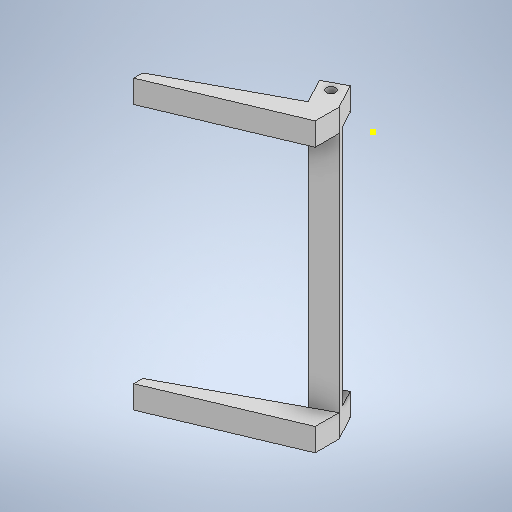
# Autodesk Inventor part: Part8
Saved by Autodesk Inventor 2025.2 (Build 292293000, 293)
## iProperties
Created: 2025-06-06
Part Number: Part8
Material: Generic
Document SubType Name: Sheet Metal
Designer: ziyuz
Density: 1 g/cm^3
Sheet Metal Rule: Default_mm
Appearance: Default
Author: ziyuz
Autodesk Inventor part; units mm, degrees
ref_plane "YZ Plane" through (0, 0, 0) normal (1, 0, 0) x (0, 1, 0)
ref_plane "XZ Plane" through (0, 0, 0) normal (0, 1, 0) x (-1, 0, 0)
ref_plane "XY Plane" through (0, 0, 0) normal (0, 0, 1) x (1, 0, 0)
sketch "Sketch1" plane through (0, 0, 0) normal (0, 1, 0) x (-1, 0, 0)
  line L0 (37.9657, 6.6302) -> (37.9657, 8.6302)
  line L1 (37.9657, 6.6302) -> (9.9657, -8.3698)
  line L2 (37.9657, 6.6302) -> (9.9657, -8.3698)
  line L3 (9.9657, -3.1386) -> (9.9657, -8.3698)
  line L4 (9.9657, -8.3698) -> (9.9657, -3.1386)
  line L5 (9.9657, -3.1386) -> (37.9657, 8.6302)
  line L6 (37.9657, 8.6302) -> (37.9657, 6.6302)
  point P0 (0, 0)
  point P1 (-42.0343, 11.6302)
  constraints: 14 end point, 2 collinear, 1 parallel
extrude "Extrusion1" add sketch "Sketch1" along normal blind 5
sketch "Sketch2" plane through (-37.9657, 0, 6.6302) normal (-0.4722214, 0, -0.88148) x (-0.88148, 0, 0.4722214)
  line L0 (-31.7648, 0) -> (-31.7648, 5) projected
  line L1 (-31.7648, 5) -> (-26.7648, 5)
  line L2 (-26.7648, 5) -> (-26.7648, -58)
  line L3 (-26.7648, -58) -> (-31.7648, -58)
  line L4 (-31.7648, -58) -> (-31.7648, 5)
  point P0 (-36.597, 0)
  point P1 (-31.7648, 0)
  dimension "d2" = 5
  dimension "d3" = 63
  constraints: 8 end point, 2 parallel, 1 horizontal, 1 perpendicular
  measures "d2" distance of L2.end L3.end
  measures "d3" distance of L1.end L2.end
extrude "Extrusion2" add sketch "Sketch2" along normal blind 6
pattern_linear "Rectangular Pattern1" count 2 spacing 58 along (0, -1, 0) of "Extrusion1"
sketch "Sketch3" plane through (-40.7991, 0, 1.3413) normal (-0.4722214, 0, -0.88148) x (-0.88148, 0, 0.4722214)
  line L0 (-26.7648, -53) -> (0, -53) projected
  line L1 (-29.2945, 0) -> (-31.7648, 0) projected
  line L2 (-26.7648, -53) -> (-31.7648, -53)
  line L3 (-31.7648, -53) -> (-31.7648, 0)
  line L4 (-31.7648, 0) -> (-26.7648, 0)
  line L5 (-26.7648, 0) -> (-26.7648, -53)
  point P0 (-36.597, 0)
  point P1 (-29.2945, 0)
  constraints: 8 end point, 2 parallel, 1 horizontal, 1 perpendicular
extrude "Extrusion3" cut sketch "Sketch3" against normal blind 4
sketch "Sketch4" plane through (-17.2065, 0, -11.2976) normal (0, -1, 0) x (0.88148, 0, -0.4722214)
  line L0 (5, 0) -> (0, 0) projected
  line L1 (2.5, 0) -> (2.5, 4)
  line L2 (5, 4) -> (0, 4) projected
  line L3 (2.5, 2) -> (5, 2)
  line L4 (5, 4) -> (5, 0) projected
  circle A0 centre (2.5, 2) radius 1
  point P0 (9.8322, 18.0838)
  dimension "d11" = 2
  constraints: 4 end point, 4 midpoint, 1 centre point, 1 coincident
  measures "d11" diameter of A0
extrude "Extrusion4" cut sketch "Sketch4" along normal blind 110 and the other way blind 20 contours A0 L1 | L1 L3 A0 | L3 L1 A0
sketch "Sketch5" plane through (-38.9102, 0, 4.8672) normal (-0.4722214, 0, -0.88148) x (-0.88148, 0, 0.4722214)
  point P0 (-36.597, 0)
equation "\"BendRadius\" = Thickness"
equation "\"BendReliefWidth\" = Thickness"
equation "\"BendReliefDepth\" = 0.5 * Thickness"
equation "\"CornerReliefSize\" = 4 * Thickness"
equation "\"MinimumRemnant\" = 2 * Thickness"
equation "\"TransitionRadius\" = BendRadius"
equation "\"JacobiRadiusSize\" = BendRadius"
equation "\"GapSize\" = Thickness"
equation "\"Thickness\" = 0.5"
body "Solid1"
